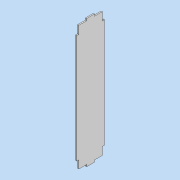
# Autodesk Inventor part: Acrly_Wand_1
Saved by Autodesk Inventor 2022 (Build 260153000, 153)
## iProperties
Created: 2021-12-15
Part Number: Acrly_Wand_1
Material: Generic
Document SubType Name: Modeling
Designer: Fabijansven
Density: 1 g/cm^3
Appearance: Default
Author: Fabijansven
Autodesk Inventor part; units mm, degrees
ref_plane "YZ Plane" through (0, 0, 0) normal (1, 0, 0) x (0, 1, 0)
ref_plane "XZ Plane" through (0, 0, 0) normal (0, 1, 0) x (-1, 0, 0)
ref_plane "XY Plane" through (0, 0, 0) normal (0, 0, 1) x (1, 0, 0)
sketch "Sketch1" plane through (0, 0, 0) normal (1, 0, 0) x (0, 1, 0)
  line L0 (0, 0) -> (522, 0)
  line L1 (522, 0) -> (522, -112)
  line L2 (522, -112) -> (0, -112)
  line L3 (0, -112) -> (0, 0)
  line L4 (522, 0) -> (514, 0)
  line L5 (514, 0) -> (514, -40)
  line L6 (514, -40) -> (522, -40)
  line L7 (522, -40) -> (522, 0)
  line L8 (522, 0) -> (482, 0)
  line L9 (482, 0) -> (482, -8)
  line L10 (482, -8) -> (522, -8)
  line L11 (522, -8) -> (522, 0)
  line L12 (856.5319, -56) -> (-65.1606, -56) construction
  line L13 (261, 165.682) -> (261, -1074.2454) construction
  line L14 (522, -112) -> (514, -112)
  line L15 (514, -112) -> (514, -72)
  line L16 (514, -72) -> (522, -72)
  line L17 (522, -72) -> (522, -112)
  line L18 (522, -112) -> (482, -112)
  line L19 (482, -112) -> (482, -104)
  line L20 (482, -104) -> (522, -104)
  line L21 (522, -104) -> (522, -112)
  line L22 (0, 0) -> (0, -112)
  line L23 (0, 0) -> (8, 0)
  line L24 (8, 0) -> (8, -40)
  line L25 (8, -40) -> (0, -40)
  line L26 (0, -40) -> (0, 0)
  line L27 (0, 0) -> (40, 0)
  line L28 (40, 0) -> (40, -8)
  line L29 (40, -8) -> (0, -8)
  line L30 (0, -8) -> (0, 0)
  line L31 (8, -72) -> (0, -72)
  line L32 (40, -104) -> (0, -104)
  line L33 (0, -112) -> (8, -112)
  line L34 (8, -112) -> (8, -72)
  line L35 (0, -72) -> (0, -112)
  line L36 (0, -112) -> (40, -112)
  line L37 (40, -112) -> (40, -104)
  line L38 (0, -104) -> (0, -112)
  point P0 (40, -112)
  point P1 (482, -112)
  point P2 (514, -104)
  point P3 (522, -72)
  point P4 (522, -40)
  point P5 (514, -8)
  point P6 (482, 0)
  point P7 (40, 0)
  point P8 (8, -8)
  point P9 (0, -40)
  point P10 (0, -72)
  point P11 (8, -104)
  dimension "d0" = 522
  dimension "d1" = 112
  dimension "d2" = 40
  dimension "d3" = 40
  dimension "d4" = 8
  dimension "d5" = 8
  dimension "d6" = 56
  dimension "d7" = 261
  constraints: 78 end point, 18 symmetric about line, 6 parallel, 4 horizontal, 3 perpendicular, 1 vertical
  measures "d0" distance of L1.end L2.end
  measures "d1" distance of L0.end L1.end
  measures "d2" distance of L4.end L5.end
  measures "d3" distance of L9.end L10.end
  measures "d4" distance of L8.end L9.end
  measures "d5" distance of L5.end L6.end
  measures "d6" distance between parallel lines of L0 L12
  measures "d7" distance between parallel lines of L3 L13
extrude "Extrusion1" add sketch "Sketch1" along normal blind 5 contours L0 L9 L10 L5 L6 L1 L16 L15 L20 L19 L2 L37 L32 L34 L31 L3 L25 L24 L29 L28
equation "\"d6\" = 0.5 * d1"
equation "\"d7\" = 0.5 * d0"
body "Solid1"
